Autodesk Inventor part; units mm, degrees
(part 5 of 6)
  spline S1198 degree 2 poles (-69.2039, -168.0401) (-69.2039, -169.0936) (-67.7114, -170.5861) (-66.6579, -170.5861) knots 0 0 0 1 2 2 2
  spline S1199 degree 2 poles (-66.6579, -170.5861) (-65.6044, -170.5861) (-64.1119, -169.0936) (-64.1119, -168.0401) knots 0 0 0 1 2 2 2
  line L962 (-64.1119, -168.0401) -> (-64.1119, -152.1497)
  spline S1200 degree 2 poles (-64.1119, -152.1497) (-64.1119, -151.7458) (-63.5676, -151.1839) (-63.1637, -151.1839) knots 0 0 0 1 2 2 2
  spline S1201 degree 2 poles (-63.1637, -151.1839) (-62.7599, -151.1839) (-62.198, -151.7458) (-62.198, -152.1497) knots 0 0 0 1 2 2 2
  line L963 (-62.198, -152.1497) -> (-62.198, -168.0401)
  spline S1202 degree 2 poles (-62.198, -168.0401) (-62.198, -169.8838) (-64.8142, -172.5) (-66.6579, -172.5) knots 0 0 0 1 2 2 2
  spline S1203 degree 2 poles (-66.6579, -172.5) (-68.5015, -172.5) (-71.1178, -169.8838) (-71.1178, -168.0401) knots 0 0 0 1 2 2 2
  line L964 (-71.1178, -168.0401) -> (-71.1178, -152.1497)
  spline S1204 degree 2 poles (-30.1552, -161.0343) (-29.7514, -161.0343) (-29.1895, -161.5962) (-29.1895, -162) knots 0 0 0 1 2 2 2
  spline S1205 degree 2 poles (-29.1895, -162) (-29.1895, -162.3863) (-29.7514, -162.9482) (-30.1552, -162.9482) knots 0 0 0 1 2 2 2
  line L965 (-30.1552, -162.9482) -> (-34.2815, -162.9482)
  line L966 (-34.2815, -162.9482) -> (-34.2815, -171.5518)
  spline S1206 degree 2 poles (-34.2815, -171.5518) (-34.2815, -171.9381) (-34.8434, -172.5) (-35.2472, -172.5) knots 0 0 0 1 2 2 2
  spline S1207 degree 2 poles (-35.2472, -172.5) (-35.6335, -172.5) (-36.1954, -171.9381) (-36.1954, -171.5518) knots 0 0 0 1 2 2 2
  line L967 (-36.1954, -171.5518) -> (-36.1954, -152.4482)
  spline S1208 degree 2 poles (-36.1954, -152.4482) (-36.1954, -152.0443) (-35.6335, -151.5) (-35.2472, -151.5) knots 0 0 0 1 2 2 2
  line L968 (-35.2472, -151.5) -> (-29.172, -151.5)
  spline S1209 degree 2 poles (-29.172, -151.5) (-28.7857, -151.5) (-28.2238, -152.0443) (-28.2238, -152.4482) knots 0 0 0 1 2 2 2
  spline S1210 degree 2 poles (-28.2238, -152.4482) (-28.2238, -152.8344) (-28.7857, -153.3963) (-29.172, -153.3963) knots 0 0 0 1 2 2 2
  line L969 (-29.172, -153.3963) -> (-34.2815, -153.3963)
  line L970 (-34.2815, -153.3963) -> (-34.2815, -161.0343)
  line L971 (-34.2815, -161.0343) -> (-30.1552, -161.0343)
  spline S1211 degree 2 poles (-0.9569, -152.4482) (-0.9569, -152.0443) (-0.3951, -151.5) (-0.0088, -151.5) knots 0 0 0 1 2 2 2
  spline S1212 degree 2 poles (-0.0088, -151.5) (0.3951, -151.5) (0.9569, -152.0443) (0.9569, -152.4482) knots 0 0 0 1 2 2 2
  line L972 (0.9569, -152.4482) -> (0.9569, -171.5518)
  spline S1213 degree 2 poles (0.9569, -171.5518) (0.9569, -171.9381) (0.3951, -172.5) (-0.0088, -172.5) knots 0 0 0 1 2 2 2
  spline S1214 degree 2 poles (-0.0088, -172.5) (-0.3951, -172.5) (-0.9569, -171.9381) (-0.9569, -171.5518) knots 0 0 0 1 2 2 2
  line L973 (-0.9569, -171.5518) -> (-0.9569, -152.4482)
  spline S1215 degree 2 poles (29.8392, -171.5518) (29.8392, -171.9381) (29.2773, -172.5) (28.8735, -172.5) knots 0 0 0 1 2 2 2
  spline S1216 degree 2 poles (28.8735, -172.5) (28.4872, -172.5) (27.9253, -171.9381) (27.9253, -171.5518) knots 0 0 0 1 2 2 2
  line L974 (27.9253, -171.5518) -> (27.9253, -152.4306)
  spline S1217 degree 2 poles (27.9253, -152.4306) (27.9253, -152.0268) (28.4872, -151.4824) (28.8735, -151.4824) knots 0 0 0 1 2 2 2
  spline S1218 degree 2 poles (28.8735, -151.4824) (29.2773, -151.4824) (29.5583, -151.7458) knots 0 0 0 1 1 1
  spline S1219 degree 2 poles (29.5583, -151.7458) (29.6636, -151.8512) (29.7163, -151.9741) knots 0 0 0 1 1 1
  line L975 (29.7163, -151.9741) -> (36.845, -167.2676)
  line L976 (36.845, -167.2676) -> (36.845, -152.4306)
  spline S1220 degree 2 poles (36.845, -152.4306) (36.845, -152.0268) (37.3894, -151.4824) (37.7932, -151.4824) knots 0 0 0 1 2 2 2
  spline S1221 degree 2 poles (37.7932, -151.4824) (38.197, -151.4824) (38.7414, -152.0268) (38.7414, -152.4306) knots 0 0 0 1 2 2 2
  line L977 (38.7414, -152.4306) -> (38.7414, -171.5694)
  spline S1222 degree 2 poles (38.7414, -171.5694) (38.7414, -171.9381) (38.478, -172.2191) knots 0 0 0 1 1 1
  spline S1223 degree 2 poles (38.478, -172.2191) (38.197, -172.5) (37.7932, -172.5) knots 0 0 0 1 1 1
  spline S1224 degree 2 poles (37.7932, -172.5) (37.3894, -172.5) (37.126, -172.2191) knots 0 0 0 1 1 1
  spline S1225 degree 2 poles (37.126, -172.2191) (36.9855, -172.0786) (36.8802, -171.8679) knots 0 0 0 1 1 1
  line L978 (36.8802, -171.8679) -> (29.8392, -156.6271)
  line L979 (29.8392, -156.6271) -> (29.8392, -171.5518)
  spline S1226 degree 2 poles (66.6754, -166.1789) (67.0617, -166.1789) (67.6236, -166.7408) (67.6236, -167.1446) knots 0 0 0 1 2 2 2
  spline S1227 degree 2 poles (67.6236, -167.1446) (67.6236, -167.5309) (67.0617, -168.0928) (66.6754, -168.0928) knots 0 0 0 1 2 2 2
  line L980 (66.6754, -168.0928) -> (63.4974, -168.0928)
  line L981 (63.4974, -168.0928) -> (62.5316, -171.7099)
  spline S1228 degree 2 poles (62.5316, -171.7099) (62.4438, -172.0084) (62.2507, -172.2191) knots 0 0 0 1 1 1
  spline S1229 degree 2 poles (62.2507, -172.2191) (61.9698, -172.5) (61.5835, -172.5) knots 0 0 0 1 1 1
  spline S1230 degree 2 poles (61.5835, -172.5) (61.1796, -172.5) (60.6178, -171.9381) (60.6178, -171.5518) knots 0 0 0 1 2 2 2
  spline S1231 degree 2 poles (60.6178, -171.5518) (60.6178, -171.4289) (60.6353, -171.3411) knots 0 0 0 1 1 1
  line L982 (60.6353, -171.3411) -> (65.7273, -152.3428)
  spline S1232 degree 2 poles (65.7273, -152.3428) (65.7975, -152.0268) (66.0082, -151.7985) knots 0 0 0 1 1 1
  spline S1233 degree 2 poles (66.0082, -151.7985) (66.2892, -151.5) (66.6754, -151.5) knots 0 0 0 1 1 1
  spline S1234 degree 2 poles (66.6754, -151.5) (67.0617, -151.5) (67.3602, -151.7985) knots 0 0 0 1 1 1
  spline S1235 degree 2 poles (67.3602, -151.7985) (67.5358, -152.0268) (67.606, -152.3428) knots 0 0 0 1 1 1
  line L983 (67.606, -152.3428) -> (72.698, -171.3411)
  spline S1236 degree 2 poles (72.698, -171.3411) (72.7156, -171.4289) (72.7156, -171.5518) knots 0 0 0 1 1 1
  spline S1237 degree 2 poles (72.7156, -171.5518) (72.7156, -171.9381) (72.1537, -172.5) (71.7674, -172.5) knots 0 0 0 1 2 2 2
  spline S1238 degree 2 poles (71.7674, -172.5) (71.3636, -172.5) (71.1002, -172.2191) knots 0 0 0 1 1 1
  spline S1239 degree 2 poles (71.1002, -172.2191) (70.8895, -172.0084) (70.8017, -171.7099) knots 0 0 0 1 1 1
  line L984 (70.8017, -171.7099) -> (66.6754, -156.2057)
  line L985 (66.6754, -156.2057) -> (64.0065, -166.1789)
  line L986 (64.0065, -166.1789) -> (66.6754, -166.1789)
  spline S1240 degree 2 poles (95.5489, -152.1497) (95.5489, -151.7458) (96.1108, -151.1839) (96.4971, -151.1839) knots 0 0 0 1 2 2 2
  spline S1241 degree 2 poles (96.4971, -151.1839) (96.9009, -151.1839) (97.4628, -151.7458) (97.4628, -152.1497) knots 0 0 0 1 2 2 2
  line L987 (97.4628, -152.1497) -> (97.4628, -168.0401)
  spline S1242 degree 2 poles (97.4628, -168.0401) (97.4628, -169.0936) (98.9553, -170.5861) (100.0088, -170.5861) knots 0 0 0 1 2 2 2
  spline S1243 degree 2 poles (100.0088, -170.5861) (101.0623, -170.5861) (102.5548, -169.0936) (102.5548, -168.0401) knots 0 0 0 1 2 2 2
  line L988 (102.5548, -168.0401) -> (102.5548, -152.1497)
  spline S1244 degree 2 poles (102.5548, -152.1497) (102.5548, -151.7458) (103.0991, -151.1839) (103.5029, -151.1839) knots 0 0 0 1 2 2 2
  spline S1245 degree 2 poles (103.5029, -151.1839) (103.9068, -151.1839) (104.4686, -151.7458) (104.4686, -152.1497) knots 0 0 0 1 2 2 2
  line L989 (104.4686, -152.1497) -> (104.4686, -168.0401)
  spline S1246 degree 2 poles (104.4686, -168.0401) (104.4686, -169.8838) (101.8524, -172.5) (100.0088, -172.5) knots 0 0 0 1 2 2 2
  spline S1247 degree 2 poles (100.0088, -172.5) (98.1651, -172.5) (95.5489, -169.8838) (95.5489, -168.0401) knots 0 0 0 1 2 2 2
  line L990 (95.5489, -168.0401) -> (95.5489, -152.1497)
  spline S1248 degree 2 poles (128.5574, -152.4482) (128.5574, -152.0443) (129.1193, -151.5) (129.5056, -151.5) knots 0 0 0 1 2 2 2
  spline S1249 degree 2 poles (129.5056, -151.5) (129.9094, -151.5) (130.4713, -152.0443) (130.4713, -152.4482) knots 0 0 0 1 2 2 2
  line L991 (130.4713, -152.4482) -> (130.4713, -161.0343)
  line L992 (130.4713, -161.0343) -> (136.1778, -161.0343)
  line L993 (136.1778, -161.0343) -> (136.1778, -152.4482)
  spline S1250 degree 2 poles (136.1778, -152.4482) (136.1778, -152.0443) (136.7397, -151.5) (137.1435, -151.5) knots 0 0 0 1 2 2 2
  spline S1251 degree 2 poles (137.1435, -151.5) (137.5298, -151.5) (138.0917, -152.0443) (138.0917, -152.4482) knots 0 0 0 1 2 2 2
  line L994 (138.0917, -152.4482) -> (138.0917, -171.5518)
  spline S1252 degree 2 poles (138.0917, -171.5518) (138.0917, -171.9381) (137.5298, -172.5) (137.1435, -172.5) knots 0 0 0 1 2 2 2
  spline S1253 degree 2 poles (137.1435, -172.5) (136.7397, -172.5) (136.1778, -171.9381) (136.1778, -171.5518) knots 0 0 0 1 2 2 2
  line L995 (136.1778, -171.5518) -> (136.1778, -162.9482)
  line L996 (136.1778, -162.9482) -> (130.4713, -162.9482)
  line L997 (130.4713, -162.9482) -> (130.4713, -171.5518)
  spline S1254 degree 2 poles (130.4713, -171.5518) (130.4713, -171.9381) (129.9094, -172.5) (129.5056, -172.5) knots 0 0 0 1 2 2 2
  spline S1255 degree 2 poles (129.5056, -172.5) (129.1193, -172.5) (128.5574, -171.9381) (128.5574, -171.5518) knots 0 0 0 1 2 2 2
  line L998 (128.5574, -171.5518) -> (128.5574, -152.4482)
  spline S1256 degree 2 poles (168.1504, -163.8436) (168.5893, -163.7207) (168.9756, -163.352) knots 0 0 0 1 1 1
  spline S1257 degree 2 poles (168.9756, -163.352) (169.5375, -162.7901) (169.5375, -162) knots 0 0 0 1 1 1
  line L999 (169.5375, -162) -> (169.5375, -155.3102)
  spline S1258 degree 2 poles (169.5375, -155.3102) (169.5375, -154.5201) (168.4137, -153.3963) (167.6236, -153.3963) knots 0 0 0 1 2 2 2
  line L1000 (167.6236, -153.3963) -> (164.4455, -153.3963)
  line L1001 (164.4455, -153.3963) -> (164.4455, -171.5518)
  spline S1259 degree 2 poles (164.4455, -171.5518) (164.4455, -171.9381) (163.8836, -172.5) (163.4798, -172.5) knots 0 0 0 1 2 2 2
  spline S1260 degree 2 poles (163.4798, -172.5) (163.0935, -172.5) (162.5316, -171.9381) (162.5316, -171.5518) knots 0 0 0 1 2 2 2
  line L1002 (162.5316, -171.5518) -> (162.5316, -152.4482)
  spline S1261 degree 2 poles (162.5316, -152.4482) (162.5316, -152.0443) (163.0935, -151.5) (163.4798, -151.5) knots 0 0 0 1 2 2 2
  line L1003 (163.4798, -151.5) -> (167.6236, -151.5)
  spline S1262 degree 2 poles (167.6236, -151.5) (169.2039, -151.5) (171.4514, -153.7299) (171.4514, -155.3102) knots 0 0 0 1 2 2 2
  line L1004 (171.4514, -155.3102) -> (171.4514, -162)
  spline S1263 degree 2 poles (171.4514, -162) (171.4514, -163.5627) (170.3276, -164.6865) knots 0 0 0 1 1 1
  spline S1264 degree 2 poles (170.3276, -164.6865) (169.9764, -165.0376) (169.5902, -165.2659) knots 0 0 0 1 1 1
  line L1005 (169.5902, -165.2659) -> (171.9781, -171.1304)
  spline S1265 degree 2 poles (171.9781, -171.1304) (172.0835, -171.3411) (172.0835, -171.5518) knots 0 0 0 1 1 1
  spline S1266 degree 2 poles (172.0835, -171.5518) (172.0835, -171.6923) (172.0308, -171.8328) knots 0 0 0 1 1 1
  spline S1267 degree 2 poles (172.0308, -171.8328) (171.9079, -172.2191) (171.5567, -172.3946) knots 0 0 0 1 1 1
  spline S1268 degree 2 poles (171.5567, -172.3946) (171.346, -172.5) (171.1353, -172.5) knots 0 0 0 1 1 1
  spline S1269 degree 2 poles (171.1353, -172.5) (170.9773, -172.5) (170.8368, -172.4649) knots 0 0 0 1 1 1
  spline S1270 degree 2 poles (170.8368, -172.4649) (170.4505, -172.342) (170.2749, -171.9732) knots 0 0 0 1 1 1
  line L1006 (170.2749, -171.9732) -> (167.5534, -165.2308)
  spline S1271 degree 2 poles (167.5534, -165.2308) (167.4305, -165.0201) (167.4305, -164.7567) knots 0 0 0 1 1 1
  spline S1272 degree 2 poles (167.4305, -164.7567) (167.4305, -164.3704) (167.729, -164.0719) knots 0 0 0 1 1 1
  spline S1273 degree 2 poles (167.729, -164.0719) (167.9045, -163.8963) (168.1504, -163.8436) knots 0 0 0 1 1 1
  spline S1274 degree 2 poles (-136.8802, 152.9749) (-137.1787, 153.3261) (-137.1787, 153.7299) knots 0 0 0 1 1 1
  spline S1275 degree 2 poles (-137.1787, 153.7299) (-137.1435, 154.1338) (-136.8626, 154.3972) knots 0 0 0 1 1 1
  spline S1276 degree 2 poles (-136.8626, 154.3972) (-136.5992, 154.643) (-136.1778, 154.643) knots 0 0 0 1 1 1
  spline S1277 degree 2 poles (-136.1778, 154.643) (-135.7915, 154.6079) (-135.4579, 154.2742) knots 0 0 0 1 1 1
  spline S1278 degree 2 poles (-135.4579, 154.2742) (-134.7556, 153.4841) (-133.7021, 153.4314) knots 0 0 0 1 1 1
  line L1007 (-133.7021, 153.4314) -> (-133.5792, 153.4314)
  spline S1279 degree 2 poles (-133.5792, 153.4314) (-132.5959, 153.4314) (-131.876, 154.0987) knots 0 0 0 1 1 1
  spline S1280 degree 2 poles (-131.876, 154.0987) (-131.0858, 154.801) (-131.0332, 155.837) knots 0 0 0 1 1 1
  line L1008 (-131.0332, 155.837) -> (-131.0332, 156.0477)
  spline S1281 degree 2 poles (-131.0332, 156.0477) (-131.0332, 158.6814) (-134.2288, 162.2107) knots 0 0 0 1 1 1
  spline S1282 degree 2 poles (-134.2288, 162.2107) (-137.4069, 165.7224) (-137.4069, 168.6722) knots 0 0 0 1 1 1
  line L1009 (-137.4069, 168.6722) -> (-137.4069, 168.9356)
  spline S1283 degree 2 poles (-137.4069, 168.9356) (-137.3016, 170.7968) (-135.932, 172.0259) knots 0 0 0 1 1 1
  spline S1284 degree 2 poles (-135.932, 172.0259) (-134.6502, 173.1672) (-132.9822, 173.1672) knots 0 0 0 1 1 1
  line L1010 (-132.9822, 173.1672) -> (-132.7188, 173.1672)
  spline S1285 degree 2 poles (-132.7188, 173.1672) (-130.8576, 173.0619) (-129.646, 171.6923) knots 0 0 0 1 1 1
  spline S1286 degree 2 poles (-129.646, 171.6923) (-129.33, 171.3411) (-129.33, 170.9548) knots 0 0 0 1 1 1
  spline S1287 degree 2 poles (-129.33, 170.9548) (-129.3651, 170.551) (-129.6636, 170.2876) knots 0 0 0 1 1 1
  spline S1288 degree 2 poles (-129.6636, 170.2876) (-129.927, 170.0418) (-130.2957, 170.0418) knots 0 0 0 1 1 1
  spline S1289 degree 2 poles (-130.2957, 170.0418) (-130.7347, 170.0594) (-131.0332, 170.4105) knots 0 0 0 1 1 1
  spline S1290 degree 2 poles (-131.0332, 170.4105) (-131.7706, 171.1831) (-132.8241, 171.2358) knots 0 0 0 1 1 1
  line L1011 (-132.8241, 171.2358) -> (-132.9997, 171.2358)
  spline S1291 degree 2 poles (-132.9997, 171.2358) (-133.9303, 171.2358) (-134.6502, 170.6037) knots 0 0 0 1 1 1
  spline S1292 degree 2 poles (-134.6502, 170.6037) (-135.4404, 169.8838) (-135.493, 168.8303) knots 0 0 0 1 1 1
  line L1012 (-135.493, 168.8303) -> (-135.493, 168.6898)
  spline S1293 degree 2 poles (-135.493, 168.6898) (-135.493, 166.4774) (-132.2623, 162.9306) knots 0 0 0 1 1 1
  spline S1294 degree 2 poles (-132.2623, 162.9306) (-129.1017, 159.4189) (-129.1017, 156.1003) knots 0 0 0 1 1 1
  spline S1295 degree 2 poles (-129.1017, 156.1003) (-129.1017, 155.9247) (-129.1193, 155.7492) knots 0 0 0 1 1 1
  spline S1296 degree 2 poles (-129.1193, 155.7492) (-129.2246, 153.888) (-130.5942, 152.6413) knots 0 0 0 1 1 1
  spline S1297 degree 2 poles (-130.5942, 152.6413) (-131.876, 151.5) (-133.5616, 151.5) knots 0 0 0 1 1 1
  line L1013 (-133.5616, 151.5) -> (-133.8074, 151.5)
  spline S1298 degree 2 poles (-133.8074, 151.5) (-135.6511, 151.6054) (-136.8802, 152.9749) knots 0 0 0 1 1 1
  spline S1299 degree 2 poles (-169.8448, 27.5518) (-169.8448, 27.9557) (-169.2829, 28.5) (-168.8966, 28.5) knots 0 0 0 1 2 2 2
  line L1014 (-168.8966, 28.5) -> (-162.8213, 28.5)
  spline S1300 degree 2 poles (-162.8213, 28.5) (-162.4351, 28.5) (-161.8732, 27.9557) (-161.8732, 27.5518) knots 0 0 0 1 2 2 2
  spline S1301 degree 2 poles (-161.8732, 27.5518) (-161.8732, 27.1656) (-162.4351, 26.6037) (-162.8213, 26.6037) knots 0 0 0 1 2 2 2
  line L1015 (-162.8213, 26.6037) -> (-167.9309, 26.6037)
  line L1016 (-167.9309, 26.6037) -> (-167.9309, 18.9657)
  line L1017 (-167.9309, 18.9657) -> (-163.8046, 18.9657)
  spline S1302 degree 2 poles (-163.8046, 18.9657) (-163.4008, 18.9657) (-162.8389, 18.4038) (-162.8389, 18) knots 0 0 0 1 2 2 2
  spline S1303 degree 2 poles (-162.8389, 18) (-162.8389, 17.6137) (-163.4008, 17.0518) (-163.8046, 17.0518) knots 0 0 0 1 2 2 2
  line L1018 (-163.8046, 17.0518) -> (-167.9309, 17.0518)
  line L1019 (-167.9309, 17.0518) -> (-167.9309, 9.4139)
  line L1020 (-167.9309, 9.4139) -> (-162.8213, 9.4139)
  spline S1304 degree 2 poles (-162.8213, 9.4139) (-162.4351, 9.4139) (-161.8732, 8.852) (-161.8732, 8.4482) knots 0 0 0 1 2 2 2
  spline S1305 degree 2 poles (-161.8732, 8.4482) (-161.8732, 8.0794) (-162.4351, 7.5) (-162.8213, 7.5) knots 0 0 0 1 2 2 2
  line L1021 (-162.8213, 7.5) -> (-168.8966, 7.5)
  spline S1306 degree 2 poles (-168.8966, 7.5) (-169.2829, 7.5) (-169.8448, 8.0619) (-169.8448, 8.4482) knots 0 0 0 1 2 2 2
  line L1022 (-169.8448, 8.4482) -> (-169.8448, 27.5518)
  spline S1307 degree 2 poles (-134.2903, 27.5518) (-134.2903, 27.9557) (-133.7284, 28.5) (-133.3421, 28.5) knots 0 0 0 1 2 2 2
  spline S1308 degree 2 poles (-133.3421, 28.5) (-132.9383, 28.5) (-132.3764, 27.9557) (-132.3764, 27.5518) knots 0 0 0 1 2 2 2
  line L1023 (-132.3764, 27.5518) -> (-132.3764, 8.4482)
  spline S1309 degree 2 poles (-132.3764, 8.4482) (-132.3764, 8.0619) (-132.9383, 7.5) (-133.3421, 7.5) knots 0 0 0 1 2 2 2
  spline S1310 degree 2 poles (-133.3421, 7.5) (-133.7284, 7.5) (-134.2903, 8.0619) (-134.2903, 8.4482) knots 0 0 0 1 2 2 2
  line L1024 (-134.2903, 8.4482) -> (-134.2903, 27.5518)
  spline S1311 degree 2 poles (-103.5468, 8.9749) (-103.8453, 9.3261) (-103.8453, 9.7299) knots 0 0 0 1 1 1
  spline S1312 degree 2 poles (-103.8453, 9.7299) (-103.8102, 10.1338) (-103.5293, 10.3972) knots 0 0 0 1 1 1
  spline S1313 degree 2 poles (-103.5293, 10.3972) (-103.2659, 10.643) (-102.8445, 10.643) knots 0 0 0 1 1 1
  spline S1314 degree 2 poles (-102.8445, 10.643) (-102.4582, 10.6079) (-102.1246, 10.2742) knots 0 0 0 1 1 1
  spline S1315 degree 2 poles (-102.1246, 10.2742) (-101.4222, 9.4841) (-100.3687, 9.4314) knots 0 0 0 1 1 1
  line L1025 (-100.3687, 9.4314) -> (-100.2458, 9.4314)
  spline S1316 degree 2 poles (-100.2458, 9.4314) (-99.2625, 9.4314) (-98.5426, 10.0987) knots 0 0 0 1 1 1
  spline S1317 degree 2 poles (-98.5426, 10.0987) (-97.7525, 10.801) (-97.6998, 11.837) knots 0 0 0 1 1 1
  line L1026 (-97.6998, 11.837) -> (-97.6998, 12.0477)
  spline S1318 degree 2 poles (-97.6998, 12.0477) (-97.6998, 14.6814) (-100.8955, 18.2107) knots 0 0 0 1 1 1
  spline S1319 degree 2 poles (-100.8955, 18.2107) (-104.0736, 21.7224) (-104.0736, 24.6722) knots 0 0 0 1 1 1
  line L1027 (-104.0736, 24.6722) -> (-104.0736, 24.9356)
  spline S1320 degree 2 poles (-104.0736, 24.9356) (-103.9682, 26.7968) (-102.5987, 28.0259) knots 0 0 0 1 1 1
  spline S1321 degree 2 poles (-102.5987, 28.0259) (-101.3169, 29.1672) (-99.6488, 29.1672) knots 0 0 0 1 1 1
  line L1028 (-99.6488, 29.1672) -> (-99.3855, 29.1672)
  spline S1322 degree 2 poles (-99.3855, 29.1672) (-97.5242, 29.0619) (-96.3127, 27.6923) knots 0 0 0 1 1 1
  spline S1323 degree 2 poles (-96.3127, 27.6923) (-95.9967, 27.3411) (-95.9967, 26.9548) knots 0 0 0 1 1 1
  spline S1324 degree 2 poles (-95.9967, 26.9548) (-96.0318, 26.551) (-96.3303, 26.2876) knots 0 0 0 1 1 1
  spline S1325 degree 2 poles (-96.3303, 26.2876) (-96.5936, 26.0418) (-96.9624, 26.0418) knots 0 0 0 1 1 1
  spline S1326 degree 2 poles (-96.9624, 26.0418) (-97.4013, 26.0594) (-97.6998, 26.4105) knots 0 0 0 1 1 1
  spline S1327 degree 2 poles (-97.6998, 26.4105) (-98.4373, 27.1831) (-99.4908, 27.2358) knots 0 0 0 1 1 1
  line L1029 (-99.4908, 27.2358) -> (-99.6664, 27.2358)
  spline S1328 degree 2 poles (-99.6664, 27.2358) (-100.597, 27.2358) (-101.3169, 26.6037) knots 0 0 0 1 1 1
  spline S1329 degree 2 poles (-101.3169, 26.6037) (-102.107, 25.8838) (-102.1597, 24.8303) knots 0 0 0 1 1 1
  line L1030 (-102.1597, 24.8303) -> (-102.1597, 24.6898)
  spline S1330 degree 2 poles (-102.1597, 24.6898) (-102.1597, 22.4774) (-98.9289, 18.9306) knots 0 0 0 1 1 1
  spline S1331 degree 2 poles (-98.9289, 18.9306) (-95.7684, 15.4189) (-95.7684, 12.1003) knots 0 0 0 1 1 1
  spline S1332 degree 2 poles (-95.7684, 12.1003) (-95.7684, 11.9247) (-95.786, 11.7492) knots 0 0 0 1 1 1
  spline S1333 degree 2 poles (-95.786, 11.7492) (-95.8913, 9.888) (-97.2609, 8.6413) knots 0 0 0 1 1 1
  spline S1334 degree 2 poles (-97.2609, 8.6413) (-98.5426, 7.5) (-100.2283, 7.5) knots 0 0 0 1 1 1
  line L1031 (-100.2283, 7.5) -> (-100.4741, 7.5)
  spline S1335 degree 2 poles (-100.4741, 7.5) (-102.3177, 7.6054) (-103.5468, 8.9749) knots 0 0 0 1 1 1
  spline S1336 degree 2 poles (-70.4417, 26.6037) (-70.8456, 26.6037) (-71.4075, 27.148) (-71.4075, 27.5518) knots 0 0 0 1 2 2 2
  spline S1337 degree 2 poles (-71.4075, 27.5518) (-71.4075, 27.9557) (-70.8456, 28.5) (-70.4417, 28.5) knots 0 0 0 1 2 2 2
  line L1032 (-70.4417, 28.5) -> (-63.1198, 28.5)
  spline S1338 degree 2 poles (-63.1198, 28.5) (-62.7336, 28.5) (-62.1717, 27.9557) (-62.1717, 27.5518) knots 0 0 0 1 2 2 2
  spline S1339 degree 2 poles (-62.1717, 27.5518) (-62.1717, 27.3587) (-62.2419, 27.1831) knots 0 0 0 1 1 1
  line L1033 (-62.2419, 27.1831) -> (-69.0546, 9.4139)
  line L1034 (-69.0546, 9.4139) -> (-63.1198, 9.4139)
  spline S1340 degree 2 poles (-63.1198, 9.4139) (-62.7336, 9.4139) (-62.1717, 8.852) (-62.1717, 8.4482) knots 0 0 0 1 2 2 2
  spline S1341 degree 2 poles (-62.1717, 8.4482) (-62.1717, 8.0794) (-62.7336, 7.5) (-63.1198, 7.5) knots 0 0 0 1 2 2 2
  line L1035 (-63.1198, 7.5) -> (-70.4417, 7.5)
  spline S1342 degree 2 poles (-70.4417, 7.5) (-70.828, 7.5) (-71.3899, 8.0794) (-71.3899, 8.4482) knots 0 0 0 1 2 2 2
  spline S1343 degree 2 poles (-71.3899, 8.4482) (-71.3899, 8.694) (-71.3021, 8.8871) knots 0 0 0 1 1 1
  line L1036 (-71.3021, 8.8871) -> (-64.5245, 26.6037)
  line L1037 (-64.5245, 26.6037) -> (-70.4417, 26.6037)
  spline S1344 degree 2 poles (-28.496, 8.3253) (-28.5486, 8.0268) (-28.7769, 7.7809) knots 0 0 0 1 1 1
  spline S1345 degree 2 poles (-28.7769, 7.7809) (-29.0578, 7.5) (-29.4441, 7.5) knots 0 0 0 1 1 1
  spline S1346 degree 2 poles (-29.4441, 7.5) (-29.848, 7.5) (-30.1113, 7.7809) knots 0 0 0 1 1 1
  spline S1347 degree 2 poles (-30.1113, 7.7809) (-30.322, 8.0268) (-30.3747, 8.3253) knots 0 0 0 1 1 1
  line L1038 (-30.3747, 8.3253) -> (-33.3421, 20.3528)
  line L1039 (-33.3421, 20.3528) -> (-36.2919, 8.3428)
  spline S1348 degree 2 poles (-36.2919, 8.3428) (-36.3446, 8.0268) (-36.5729, 7.7809) knots 0 0 0 1 1 1
  spline S1349 degree 2 poles (-36.5729, 7.7809) (-36.8538, 7.5) (-37.2401, 7.5) knots 0 0 0 1 1 1
  spline S1350 degree 2 poles (-37.2401, 7.5) (-37.644, 7.5) (-37.9073, 7.7809) knots 0 0 0 1 1 1
  spline S1351 degree 2 poles (-37.9073, 7.7809) (-38.1356, 8.0268) (-38.2058, 8.3253) knots 0 0 0 1 1 1
  line L1040 (-38.2058, 8.3253) -> (-42.7886, 27.3411)
  spline S1352 degree 2 poles (-42.7886, 27.3411) (-42.8062, 27.4465) (-42.8062, 27.5518) knots 0 0 0 1 1 1
  spline S1353 degree 2 poles (-42.8062, 27.5518) (-42.8062, 27.9557) (-42.2618, 28.5) (-41.858, 28.5) knots 0 0 0 1 2 2 2
  spline S1354 degree 2 poles (-41.858, 28.5) (-41.4542, 28.5) (-41.1732, 28.2366) knots 0 0 0 1 1 1
  spline S1355 degree 2 poles (-41.1732, 28.2366) (-40.9625, 28.0084) (-40.9098, 27.7099) knots 0 0 0 1 1 1
  line L1041 (-40.9098, 27.7099) -> (-37.2401, 12.5393)
  line L1042 (-37.2401, 12.5393) -> (-34.3605, 24.3737)
  spline S1356 degree 2 poles (-34.3605, 24.3737) (-34.2552, 24.8127) (-33.7284, 25.3219) (-33.3246, 25.3219) knots 0 0 0 1 2 2 2
  spline S1357 degree 2 poles (-33.3246, 25.3219) (-32.9207, 25.3219) (-32.4115, 24.7776) (-32.3237, 24.3737) knots 0 0 0 1 2 2 2
  line L1043 (-32.3237, 24.3737) -> (-29.4441, 12.5393)
  line L1044 (-29.4441, 12.5393) -> (-25.7744, 27.7099)
  spline S1358 degree 2 poles (-25.7744, 27.7099) (-25.7217, 28.0084) (-25.4935, 28.2366) knots 0 0 0 1 1 1
  spline S1359 degree 2 poles (-25.4935, 28.2366) (-25.2301, 28.5) (-24.8262, 28.5) knots 0 0 0 1 1 1
  spline S1360 degree 2 poles (-24.8262, 28.5) (-24.4224, 28.5) (-23.8781, 27.9557) (-23.8781, 27.5518) knots 0 0 0 1 2 2 2
  spline S1361 degree 2 poles (-23.8781, 27.5518) (-23.8781, 27.4465) (-23.8956, 27.3411) knots 0 0 0 1 1 1
  line L1045 (-23.8956, 27.3411) -> (-28.496, 8.3253)
  spline S1362 degree 2 poles (-2.467, 28.3595) (-2.2212, 28.5176) (-1.9051, 28.5176) knots 0 0 0 1 1 1
  spline S1363 degree 2 poles (-1.9051, 28.5176) (-1.5188, 28.5176) (-0.9569, 27.9557) (-0.9569, 27.5694) knots 0 0 0 1 2 2 2
  spline S1364 degree 2 poles (-0.9569, 27.5694) (-0.9569, 27.1656) (-1.2203, 26.9022) knots 0 0 0 1 1 1
  spline S1365 degree 2 poles (-1.2203, 26.9022) (-1.3081, 26.8319) (-1.3783, 26.7617) knots 0 0 0 1 1 1
  spline S1366 degree 2 poles (-1.3783, 26.7617) (-1.6066, 26.6212) (-1.7997, 26.4281) knots 0 0 0 1 1 1
  spline S1367 degree 2 poles (-1.7997, 26.4281) (-2.5372, 25.6731) (-2.5372, 24.6196) knots 0 0 0 1 1 1
  line L1046 (-2.5372, 24.6196) -> (-2.5372, 11.398)
  spline S1368 degree 2 poles (-2.5372, 11.398) (-2.5372, 10.3445) (-1.7997, 9.607) knots 0 0 0 1 1 1
  spline S1369 degree 2 poles (-1.7997, 9.607) (-1.6066, 9.4139) (-1.3783, 9.2734) knots 0 0 0 1 1 1
  spline S1370 degree 2 poles (-1.3783, 9.2734) (-1.3081, 9.2207) (-1.2379, 9.1505) knots 0 0 0 1 1 1
  spline S1371 degree 2 poles (-1.2379, 9.1505) (-0.9569, 8.8696) (-0.9569, 8.4657) knots 0 0 0 1 1 1
  spline S1372 degree 2 poles (-0.9569, 8.4657) (-0.9569, 8.0794) (-1.5188, 7.5176) (-1.9051, 7.5176) knots 0 0 0 1 2 2 2
  spline S1373 degree 2 poles (-1.9051, 7.5176) (-2.2036, 7.5176) (-2.4319, 7.658) knots 0 0 0 1 1 1
  spline S1374 degree 2 poles (-2.4319, 7.658) (-2.8181, 7.9214) (-3.1518, 8.255) knots 0 0 0 1 1 1
  spline S1375 degree 2 poles (-3.1518, 8.255) (-4.4511, 9.5543) (-4.4511, 11.398) knots 0 0 0 1 1 1
  line L1047 (-4.4511, 11.398) -> (-4.4511, 24.6196)
  spline S1376 degree 2 poles (-4.4511, 24.6196) (-4.4511, 26.4808) (-3.1518, 27.7801) knots 0 0 0 1 1 1
  spline S1377 degree 2 poles (-3.1518, 27.7801) (-2.8181, 28.1137) (-2.467, 28.3595) knots 0 0 0 1 1 1
  spline S1378 degree 2 poles (1.5013, 26.6915) (1.3608, 26.7617) (1.2379, 26.8846) knots 0 0 0 1 1 1
  spline S1379 degree 2 poles (1.2379, 26.8846) (0.9569, 27.1656) (0.9569, 27.5518) knots 0 0 0 1 1 1
  spline S1380 degree 2 poles (0.9569, 27.5518) (0.9569, 27.9557) (1.5188, 28.5176) (1.9051, 28.5176) knots 0 0 0 1 2 2 2
  spline S1381 degree 2 poles (1.9051, 28.5176) (2.2212, 28.5176) (2.4845, 28.342) knots 0 0 0 1 1 1
  spline S1382 degree 2 poles (2.4845, 28.342) (2.8357, 28.0962) (3.1518, 27.7801) knots 0 0 0 1 1 1
  spline S1383 degree 2 poles (3.1518, 27.7801) (4.4511, 26.4808) (4.4511, 24.6196) knots 0 0 0 1 1 1
  line L1048 (4.4511, 24.6196) -> (4.4511, 11.398)
  spline S1384 degree 2 poles (4.4511, 11.398) (4.4511, 9.5543) (3.1518, 8.255) knots 0 0 0 1 1 1
  spline S1385 degree 2 poles (3.1518, 8.255) (2.8006, 7.9038) (2.4143, 7.6405) knots 0 0 0 1 1 1
  spline S1386 degree 2 poles (2.4143, 7.6405) (2.2036, 7.5) (1.9051, 7.5) knots 0 0 0 1 1 1
  spline S1387 degree 2 poles (1.9051, 7.5) (1.5188, 7.5) (0.9569, 8.0794) (0.9569, 8.4482) knots 0 0 0 1 2 2 2
  spline S1388 degree 2 poles (0.9569, 8.4482) (0.9569, 8.852) (1.2379, 9.1329) knots 0 0 0 1 1 1
  spline S1389 degree 2 poles (1.2379, 9.1329) (1.3081, 9.2032) (1.3783, 9.2559) knots 0 0 0 1 1 1
  spline S1390 degree 2 poles (1.3783, 9.2559) (1.589, 9.3963) (1.7997, 9.607) knots 0 0 0 1 1 1
  spline S1391 degree 2 poles (1.7997, 9.607) (2.5548, 10.3445) (2.5548, 11.398) knots 0 0 0 1 1 1
  line L1049 (2.5548, 11.398) -> (2.5548, 24.6196)
  spline S1392 degree 2 poles (2.5548, 24.6196) (2.5548, 25.6731) (1.7997, 26.4281) knots 0 0 0 1 1 1
  spline S1393 degree 2 poles (1.7997, 26.4281) (1.6593, 26.5686) (1.5013, 26.6915) knots 0 0 0 1 1 1
  spline S1394 degree 2 poles (-2.3089, 33.6271) (-1.7822, 33.6271) (-1.0272, 32.8721) (-1.0272, 32.3453) knots 0 0 0 1 2 2 2
  spline S1395 degree 2 poles (-1.0272, 32.3453) (-1.0272, 31.8186) (-1.7822, 31.0811) (-2.3089, 31.0811) knots 0 0 0 1 2 2 2
  spline S1396 degree 2 poles (-2.3089, 31.0811) (-2.8357, 31.0811) (-3.5732, 31.8186) (-3.5732, 32.3453) knots 0 0 0 1 2 2 2
  spline S1397 degree 2 poles (-3.5732, 32.3453) (-3.5732, 32.8721) (-2.8357, 33.6271) (-2.3089, 33.6271) knots 0 0 0 1 2 2 2
  spline S1398 degree 2 poles (2.3265, 33.6271) (2.8533, 33.6271) (3.5907, 32.8721) (3.5907, 32.3453) knots 0 0 0 1 2 2 2
  spline S1399 degree 2 poles (3.5907, 32.3453) (3.5907, 31.8186) (2.8533, 31.0811) (2.3265, 31.0811) knots 0 0 0 1 2 2 2
  spline S1400 degree 2 poles (2.3265, 31.0811) (1.7997, 31.0811) (1.0447, 31.8186) (1.0447, 32.3453) knots 0 0 0 1 2 2 2
  spline S1401 degree 2 poles (1.0447, 32.3453) (1.0447, 32.8721) (1.7997, 33.6271) (2.3265, 33.6271) knots 0 0 0 1 2 2 2
  spline S1402 degree 2 poles (32.3764, 27.5518) (32.3764, 27.9557) (32.9383, 28.5) (33.3246, 28.5) knots 0 0 0 1 2 2 2
  spline S1403 degree 2 poles (33.3246, 28.5) (33.7284, 28.5) (34.2903, 27.9557) (34.2903, 27.5518) knots 0 0 0 1 2 2 2
  line L1050 (34.2903, 27.5518) -> (34.2903, 8.4482)
  spline S1404 degree 2 poles (34.2903, 8.4482) (34.2903, 8.0619) (33.7284, 7.5) (33.3246, 7.5) knots 0 0 0 1 2 2 2
  spline S1405 degree 2 poles (33.3246, 7.5) (32.9383, 7.5) (32.3764, 8.0619) (32.3764, 8.4482) knots 0 0 0 1 2 2 2
  line L1051 (32.3764, 8.4482) -> (32.3764, 27.5518)
  spline S1406 degree 2 poles (63.1198, 8.9749) (62.8213, 9.3261) (62.8213, 9.7299) knots 0 0 0 1 1 1
  spline S1407 degree 2 poles (62.8213, 9.7299) (62.8565, 10.1338) (63.1374, 10.3972) knots 0 0 0 1 1 1
  spline S1408 degree 2 poles (63.1374, 10.3972) (63.4008, 10.643) (63.8222, 10.643) knots 0 0 0 1 1 1
  spline S1409 degree 2 poles (63.8222, 10.643) (64.2085, 10.6079) (64.5421, 10.2742) knots 0 0 0 1 1 1
  spline S1410 degree 2 poles (64.5421, 10.2742) (65.2444, 9.4841) (66.2979, 9.4314) knots 0 0 0 1 1 1
  line L1052 (66.2979, 9.4314) -> (66.4208, 9.4314)
  spline S1411 degree 2 poles (66.4208, 9.4314) (67.4041, 9.4314) (68.124, 10.0987) knots 0 0 0 1 1 1
  spline S1412 degree 2 poles (68.124, 10.0987) (68.9142, 10.801) (68.9668, 11.837) knots 0 0 0 1 1 1
  line L1053 (68.9668, 11.837) -> (68.9668, 12.0477)
  spline S1413 degree 2 poles (68.9668, 12.0477) (68.9668, 14.6814) (65.7712, 18.2107) knots 0 0 0 1 1 1
  spline S1414 degree 2 poles (65.7712, 18.2107) (62.5931, 21.7224) (62.5931, 24.6722) knots 0 0 0 1 1 1
  line L1054 (62.5931, 24.6722) -> (62.5931, 24.9356)
  spline S1415 degree 2 poles (62.5931, 24.9356) (62.6984, 26.7968) (64.068, 28.0259) knots 0 0 0 1 1 1
  spline S1416 degree 2 poles (64.068, 28.0259) (65.3498, 29.1672) (67.0178, 29.1672) knots 0 0 0 1 1 1
  line L1055 (67.0178, 29.1672) -> (67.2812, 29.1672)
  spline S1417 degree 2 poles (67.2812, 29.1672) (69.1424, 29.0619) (70.354, 27.6923) knots 0 0 0 1 1 1
  spline S1418 degree 2 poles (70.354, 27.6923) (70.67, 27.3411) (70.67, 26.9548) knots 0 0 0 1 1 1
  spline S1419 degree 2 poles (70.67, 26.9548) (70.6349, 26.551) (70.3364, 26.2876) knots 0 0 0 1 1 1
  spline S1420 degree 2 poles (70.3364, 26.2876) (70.073, 26.0418) (69.7043, 26.0418) knots 0 0 0 1 1 1
  spline S1421 degree 2 poles (69.7043, 26.0418) (69.2653, 26.0594) (68.9668, 26.4105) knots 0 0 0 1 1 1
  spline S1422 degree 2 poles (68.9668, 26.4105) (68.2294, 27.1831) (67.1759, 27.2358) knots 0 0 0 1 1 1
  line L1056 (67.1759, 27.2358) -> (67.0003, 27.2358)
  spline S1423 degree 2 poles (67.0003, 27.2358) (66.0697, 27.2358) (65.3498, 26.6037) knots 0 0 0 1 1 1
  spline S1424 degree 2 poles (65.3498, 26.6037) (64.5596, 25.8838) (64.507, 24.8303) knots 0 0 0 1 1 1
  line L1057 (64.507, 24.8303) -> (64.507, 24.6898)
  spline S1425 degree 2 poles (64.507, 24.6898) (64.507, 22.4774) (67.7377, 18.9306) knots 0 0 0 1 1 1
  spline S1426 degree 2 poles (67.7377, 18.9306) (70.8983, 15.4189) (70.8983, 12.1003) knots 0 0 0 1 1 1
  spline S1427 degree 2 poles (70.8983, 12.1003) (70.8983, 11.9247) (70.8807, 11.7492) knots 0 0 0 1 1 1
  spline S1428 degree 2 poles (70.8807, 11.7492) (70.7754, 9.888) (69.4058, 8.6413) knots 0 0 0 1 1 1
  spline S1429 degree 2 poles (69.4058, 8.6413) (68.124, 7.5) (66.4384, 7.5) knots 0 0 0 1 1 1
  line L1058 (66.4384, 7.5) -> (66.1926, 7.5)
  spline S1430 degree 2 poles (66.1926, 7.5) (64.3489, 7.6054) (63.1198, 8.9749) knots 0 0 0 1 1 1
  spline S1431 degree 2 poles (100.8691, 9.4139) (101.7822, 9.4841) (102.4319, 10.1338) knots 0 0 0 1 1 1
  spline S1432 degree 2 poles (102.4319, 10.1338) (103.1869, 10.8712) (103.1869, 11.9247) knots 0 0 0 1 1 1
  line L1059 (103.1869, 11.9247) -> (103.1869, 24.0577)
  spline S1433 degree 2 poles (103.1869, 24.0577) (103.1869, 25.1112) (101.6944, 26.6037) (100.6409, 26.6037) knots 0 0 0 1 2 2 2
  line L1060 (100.6409, 26.6037) -> (98.0949, 26.6037)
  line L1061 (98.0949, 26.6037) -> (98.0949, 8.4482)
  spline S1434 degree 2 poles (98.0949, 8.4482) (98.0949, 8.0619) (97.533, 7.5) (97.1292, 7.5) knots 0 0 0 1 2 2 2
  spline S1435 degree 2 poles (97.1292, 7.5) (96.7429, 7.5) (96.181, 8.0619) (96.181, 8.4482) knots 0 0 0 1 2 2 2
  line L1062 (96.181, 8.4482) -> (96.181, 27.5518)
  spline S1436 degree 2 poles (96.181, 27.5518) (96.181, 27.9557) (96.7429, 28.5) (97.1292, 28.5) knots 0 0 0 1 2 2 2
  line L1063 (97.1292, 28.5) -> (100.6409, 28.5)
  spline S1437 degree 2 poles (100.6409, 28.5) (102.4845, 28.5) (105.1008, 25.9013) (105.1008, 24.0577) knots 0 0 0 1 2 2 2
  line L1064 (105.1008, 24.0577) -> (105.1008, 11.9247)
  spline S1438 degree 2 poles (105.1008, 11.9247) (105.1008, 10.0811) (103.7839, 8.7818) knots 0 0 0 1 1 1
  spline S1439 degree 2 poles (103.7839, 8.7818) (102.625, 7.6054) (101.0272, 7.5) knots 0 0 0 1 1 1
  spline S1440 degree 2 poles (101.0272, 7.5) (100.5531, 7.5) (100.0088, 8.0619) (100.0088, 8.4482) knots 0 0 0 1 2 2 2
  spline S1441 degree 2 poles (100.0088, 8.4482) (100.0088, 8.852) (100.2897, 9.1154) knots 0 0 0 1 1 1
  spline S1442 degree 2 poles (100.2897, 9.1154) (100.518, 9.3788) (100.8691, 9.4139) knots 0 0 0 1 1 1
  spline S1443 degree 2 poles (134.817, 16.1564) (135.256, 16.2793) (135.6423, 16.648) knots 0 0 0 1 1 1
  spline S1444 degree 2 poles (135.6423, 16.648) (136.2042, 17.2099) (136.2042, 18) knots 0 0 0 1 1 1
  line L1065 (136.2042, 18) -> (136.2042, 24.6898)
  spline S1445 degree 2 poles (136.2042, 24.6898) (136.2042, 25.4799) (135.0804, 26.6037) (134.2903, 26.6037) knots 0 0 0 1 2 2 2
  line L1066 (134.2903, 26.6037) -> (131.1122, 26.6037)
  line L1067 (131.1122, 26.6037) -> (131.1122, 8.4482)
  spline S1446 degree 2 poles (131.1122, 8.4482) (131.1122, 8.0619) (130.5503, 7.5) (130.1465, 7.5) knots 0 0 0 1 2 2 2
  spline S1447 degree 2 poles (130.1465, 7.5) (129.7602, 7.5) (129.1983, 8.0619) (129.1983, 8.4482) knots 0 0 0 1 2 2 2
  line L1068 (129.1983, 8.4482) -> (129.1983, 27.5518)
  spline S1448 degree 2 poles (129.1983, 27.5518) (129.1983, 27.9557) (129.7602, 28.5) (130.1465, 28.5) knots 0 0 0 1 2 2 2
  line L1069 (130.1465, 28.5) -> (134.2903, 28.5)
  spline S1449 degree 2 poles (134.2903, 28.5) (135.8705, 28.5) (138.118, 26.2701) (138.118, 24.6898) knots 0 0 0 1 2 2 2
  line L1070 (138.118, 24.6898) -> (138.118, 18)
  spline S1450 degree 2 poles (138.118, 18) (138.118, 16.4373) (136.9943, 15.3135) knots 0 0 0 1 1 1
  spline S1451 degree 2 poles (136.9943, 15.3135) (136.6431, 14.9624) (136.2568, 14.7341) knots 0 0 0 1 1 1
  line L1071 (136.2568, 14.7341) -> (138.6448, 8.8696)
  spline S1452 degree 2 poles (138.6448, 8.8696) (138.7501, 8.6589) (138.7501, 8.4482) knots 0 0 0 1 1 1
  spline S1453 degree 2 poles (138.7501, 8.4482) (138.7501, 8.3077) (138.6975, 8.1672) knots 0 0 0 1 1 1
  spline S1454 degree 2 poles (138.6975, 8.1672) (138.5746, 7.7809) (138.2234, 7.6054) knots 0 0 0 1 1 1
  spline S1455 degree 2 poles (138.2234, 7.6054) (138.0127, 7.5) (137.802, 7.5) knots 0 0 0 1 1 1
  spline S1456 degree 2 poles (137.802, 7.5) (137.644, 7.5) (137.5035, 7.5351) knots 0 0 0 1 1 1
  spline S1457 degree 2 poles (137.5035, 7.5351) (137.1172, 7.658) (136.9416, 8.0268) knots 0 0 0 1 1 1
  line L1072 (136.9416, 8.0268) -> (134.22, 14.7692)
  spline S1458 degree 2 poles (134.22, 14.7692) (134.0971, 14.9799) (134.0971, 15.2433) knots 0 0 0 1 1 1
  spline S1459 degree 2 poles (134.0971, 15.2433) (134.0971, 15.6296) (134.3956, 15.9281) knots 0 0 0 1 1 1
  spline S1460 degree 2 poles (134.3956, 15.9281) (134.5712, 16.1037) (134.817, 16.1564) knots 0 0 0 1 1 1
  spline S1461 degree 2 poles (162.2156, 27.8503) (162.2156, 28.2542) (162.7775, 28.8161) (163.1637, 28.8161) knots 0 0 0 1 2 2 2
  spline S1462 degree 2 poles (163.1637, 28.8161) (163.5676, 28.8161) (164.1295, 28.2542) (164.1295, 27.8503) knots 0 0 0 1 2 2 2
  line L1073 (164.1295, 27.8503) -> (164.1295, 11.9599)
  spline S1463 degree 2 poles (164.1295, 11.9599) (164.1295, 10.9064) (165.6219, 9.4139) (166.6754, 9.4139) knots 0 0 0 1 2 2 2
  spline S1464 degree 2 poles (166.6754, 9.4139) (167.729, 9.4139) (169.2214, 10.9064) (169.2214, 11.9599) knots 0 0 0 1 2 2 2
  line L1074 (169.2214, 11.9599) -> (169.2214, 27.8503)
  spline S1465 degree 2 poles (169.2214, 27.8503) (169.2214, 28.2542) (169.7657, 28.8161) (170.1696, 28.8161) knots 0 0 0 1 2 2 2
  spline S1466 degree 2 poles (170.1696, 28.8161) (170.5734, 28.8161) (171.1353, 28.2542) (171.1353, 27.8503) knots 0 0 0 1 2 2 2
  line L1075 (171.1353, 27.8503) -> (171.1353, 11.9599)
  spline S1467 degree 2 poles (171.1353, 11.9599) (171.1353, 10.1162) (168.5191, 7.5) (166.6754, 7.5) knots 0 0 0 1 2 2 2
  spline S1468 degree 2 poles (166.6754, 7.5) (164.8318, 7.5) (162.2156, 10.1162) (162.2156, 11.9599) knots 0 0 0 1 2 2 2
  line L1076 (162.2156, 11.9599) -> (162.2156, 27.8503)
  spline S1469 degree 2 poles (164.3577, 33.9256) (164.8845, 33.9256) (165.6395, 33.1706) (165.6395, 32.6438) knots 0 0 0 1 2 2 2
  spline S1470 degree 2 poles (165.6395, 32.6438) (165.6395, 32.1171) (164.8845, 31.3796) (164.3577, 31.3796) knots 0 0 0 1 2 2 2
  spline S1471 degree 2 poles (164.3577, 31.3796) (163.831, 31.3796) (163.0935, 32.1171) (163.0935, 32.6438) knots 0 0 0 1 2 2 2
  spline S1472 degree 2 poles (163.0935, 32.6438) (163.0935, 33.1706) (163.831, 33.9256) (164.3577, 33.9256) knots 0 0 0 1 2 2 2
  spline S1473 degree 2 poles (168.9932, 33.9256) (169.5199, 33.9256) (170.2749, 33.1706) (170.2749, 32.6438) knots 0 0 0 1 2 2 2
  spline S1474 degree 2 poles (170.2749, 32.6438) (170.2749, 32.1171) (169.5199, 31.3796) (168.9932, 31.3796) knots 0 0 0 1 2 2 2
  spline S1475 degree 2 poles (168.9932, 31.3796) (168.4664, 31.3796) (167.729, 32.1171) (167.729, 32.6438) knots 0 0 0 1 2 2 2
  spline S1476 degree 2 poles (167.729, 32.6438) (167.729, 33.1706) (168.4664, 33.9256) (168.9932, 33.9256) knots 0 0 0 1 2 2 2
  point P0 (0, 0)
  point P1 (166.6667, -191.8333)
  point P2 (133.3333, -191.8333)
  point P3 (100, -191.8333)
  point P4 (66.6667, -191.8333)
  point P5 (33.3333, -191.8333)
  point P6 (0, -191.8333)
  point P7 (-33.3333, -191.8333)
  point P8 (-66.6667, -191.8333)
  point P9 (-100, -191.8333)
  point P10 (-133.3333, -191.8333)
  point P11 (-166.6667, -191.8333)
  point P12 (166.6667, -155.8333)
  point P13 (133.3333, -155.8333)
  point P14 (100, -155.8333)
  point P15 (66.6667, -155.8333)
  point P16 (33.3333, -155.8333)
  point P17 (0, -155.8333)
  point P18 (-33.3333, -155.8333)
  point P19 (-66.6667, -155.8333)
  point P20 (-100, -155.8333)
  point P21 (-133.3333, -155.8333)
  point P22 (-166.6667, -155.8333)
  point P23 (166.6667, -119.8333)
  point P24 (133.3333, -119.8333)
  point P25 (100, -119.8333)
  point P26 (66.6667, -119.8333)
  point P27 (33.3333, -119.8333)
  point P28 (0, -119.8333)
  point P29 (-33.3333, -119.8333)
  point P30 (-66.6667, -119.8333)
  point P31 (-100, -119.8333)
  point P32 (-133.3333, -119.8333)
  point P33 (-166.6667, -119.8333)
  point P34 (166.6667, -83.8333)
  point P35 (133.3333, -83.8333)
  point P36 (100, -83.8333)
  point P37 (66.6667, -83.8333)
  point P38 (33.3333, -83.8333)
  point P39 (0, -83.8333)
  point P40 (-33.3333, -83.8333)
  point P41 (-66.6667, -83.8333)
  point P42 (-100, -83.8333)
  point P43 (-133.3333, -83.8333)
  point P44 (-166.6667, -83.8333)
  point P45 (166.6667, -47.8333)
  point P46 (133.3333, -47.8333)
  point P47 (100, -47.8333)
  point P48 (66.6667, -47.8333)
  point P49 (33.3333, -47.8333)
  point P50 (0, -47.8333)
  point P51 (-33.3333, -47.8333)
  point P52 (-66.6667, -47.8333)
  point P53 (-100, -47.8333)
  point P54 (-133.3333, -47.8333)
  point P55 (-166.6667, -47.8333)
  point P56 (166.6667, -11.8333)
  point P57 (133.3333, -11.8333)
  point P58 (100, -11.8333)
  point P59 (66.6667, -11.8333)
  point P60 (33.3333, -11.8333)
  point P61 (0, -11.8333)
  point P62 (-33.3333, -11.8333)
  point P63 (-66.6667, -11.8333)
  point P64 (-100, -11.8333)
  point P65 (-133.3333, -11.8333)
  point P66 (-166.6667, -11.8333)
  point P67 (166.6667, 24.1667)
  point P68 (133.3333, 24.1667)
  point P69 (100, 24.1667)
  point P70 (66.6667, 24.1667)
  point P71 (33.3333, 24.1667)
  point P72 (0, 24.1667)
  point P73 (-33.3333, 24.1667)
  point P74 (-66.6667, 24.1667)
  point P75 (-100, 24.1667)
  point P76 (-133.3333, 24.1667)
  point P77 (-166.6667, 24.1667)
  point P78 (166.6667, 60.1667)
  point P79 (133.3333, 60.1667)
  point P80 (100, 60.1667)
  point P81 (66.6667, 60.1667)
  point P82 (33.3333, 60.1667)
  point P83 (0, 60.1667)
  point P84 (-33.3333, 60.1667)
  point P85 (-66.6667, 60.1667)
  point P86 (-100, 60.1667)
  point P87 (-133.3333, 60.1667)
  point P88 (-166.6667, 60.1667)
  point P89 (166.6667, 96.1667)
  point P90 (133.3333, 96.1667)
  point P91 (100, 96.1667)
  point P92 (66.6667, 96.1667)
  point P93 (33.3333, 96.1667)
  point P94 (0, 96.1667)
  point P95 (-33.3333, 96.1667)
  point P96 (-66.6667, 96.1667)
  point P97 (-100, 96.1667)
  point P98 (-133.3333, 96.1667)
  point P99 (-166.6667, 96.1667)
  point P100 (166.6667, 132.1667)
  point P101 (133.3333, 132.1667)
  point P102 (100, 132.1667)
  point P103 (66.6667, 132.1667)
  point P104 (33.3333, 132.1667)
  point P105 (0, 132.1667)
  point P106 (-33.3333, 132.1667)
  point P107 (-66.6667, 132.1667)
  point P108 (-100, 132.1667)
  point P109 (-133.3333, 132.1667)
  point P110 (-166.6667, 132.1667)
  point P111 (166.6667, 168.1667)
  point P112 (133.3333, 168.1667)
  point P113 (100, 168.1667)
  point P114 (66.6667, 168.1667)
  point P115 (33.3333, 168.1667)
  point P116 (0, 168.1667)
  point P117 (-33.3333, 168.1667)
  point P118 (-66.6667, 168.1667)
  point P119 (-100, 168.1667)
  point P120 (-133.3333, 168.1667)
  point P121 (-166.6667, 168.1667)
  point P122 (-83.3135, 168.1667)
  point P123 (83.3532, 168.1667)
  point P124 (-16.6468, 168.1667)
  point P125 (-50, 168.1667)
  point P126 (116.6865, 168.1667)
  point P127 (16.6865, 168.1667)
  point P128 (150.0198, 168.1667)
  point P129 (50, 166.6667)
  point P130 (-183.3333, 168.1667)
  point P131 (-166.6667, 184.8333)
  point P132 (-131.4815, 148.1481)
  point P133 (-133.3333, 152.5135)
  point P134 (-116.6667, 168.1667)
  point P135 (-100, 184.8333)
  point P136 (-83.3333, 168.1667)
  point P137 (-66.6667, 184.8333)
  point P138 (-50, 168.1667)
  point P139 (-33.3333, 184.8333)
  point P140 (-16.6667, 168.1667)
  point P141 (-16.6667, 168.1667)
  point P142 (0, 184.8333)
  point P143 (16.6667, 168.1667)
  point P144 (16.6667, 168.1667)
  point P145 (33.3333, 184.8333)
  point P146 (50, 168.1667)
  point P147 (50, 168.1667)
  point P148 (66.6667, 184.8333)
  point P149 (83.3333, 168.1667)
  point P150 (0, 151.5)
  point P151 (33.3333, 151.5)
  point P152 (66.6667, 151.5)
  point P153 (83.3333, 168.1667)
  point P154 (100, 184.8333)
  point P155 (116.6667, 168.1667)
  point P156 (116.6667, 168.1667)
  point P157 (133.3333, 184.8333)
  point P158 (150, 168.1667)
  point P159 (150, 168.1667)
  point P160 (166.6667, 184.8333)
  point P161 (183.3333, 168.1667)
  point P162 (166.6667, 151.5)
  point P163 (-150, 132.1667)
  point P164 (-133.3333, 148.8333)
  point P165 (-183.3333, 132.1667)
  point P166 (-166.6667, 148.8333)
  point P167 (-133.3333, 115.5)
  point P168 (-116.6667, 132.1667)
  point P169 (-100, 148.8333)
  point P170 (-100, 115.5)
  point P171 (-83.3333, 132.1667)
  point P172 (-66.6667, 148.8333)
  point P173 (-66.6667, 115.5)
  point P174 (-50, 132.1667)
  point P175 (-33.3333, 148.8333)
  point P176 (-33.3333, 115.5)
  point P177 (-16.6667, 132.1667)
  point P178 (0, 148.8333)
  point P179 (0, 115.5)
  point P180 (-16.6667, 132.1667)
  point P181 (16.6667, 132.1667)
  point P182 (16.6667, 132.1667)
  point P183 (33.3333, 148.8333)
  point P184 (33.3333, 115.5)
  point P185 (50, 132.1667)
  point P186 (50, 132.1667)
  point P187 (66.6667, 148.8333)
  point P188 (66.6667, 115.5)
  point P189 (83.3333, 132.1667)
  point P190 (83.3333, 132.1667)
  point P191 (100, 148.8333)
  point P192 (100, 115.5)
  point P193 (116.6667, 132.1667)
  point P194 (115.3333, 133.5)
  point P195 (133.3333, 151.5)
  point P196 (151.3333, 133.5)
  point P197 (133.3333, 115.5)
  point P198 (148.6667, 133.5)
  point P199 (166.6667, 151.5)
  dimension "d83" = 16.6667
  dimension "d84" = 16.6667
  dimension "d85" = 366.6667
  dimension "d96" = 46.6667
  dimension "d106" = 33.3333
  dimension "d109" = 36
  dimension "d151" = 74.1667
  dimension "d152" = 61.8333
  constraints: 395 midpoint, 127 horizontal alignment, 124 vertical alignment, 114 collinear, 112 perpendicular, 8 end point, 2 coincident, 2 horizontal, 2 parallel, 1 vertical, 340 other
  measures "d83" distance from line of L7 point (166.667, -191.833)
  measures "d84" distance from line of point (166.667, -191.833) L4
  measures "d85" distance of L4.start L4.end
  measures "d96" distance between parallel lines of L3 L7
  measures "d106" distance of point (166.667, -191.833) point (133.333, -191.833)
  measures "d109" distance of point (166.667, -191.833) point (166.667, -155.833)
  measures "d151" distance from line of L2 point (166.667, -155.833)
  measures "d152" distance from line of L0 point (166.667, 168.167)